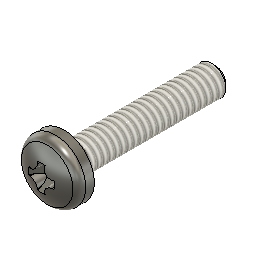
Airmote (Autodesk Fusion 360 archive; units mm, degrees)
design "Type I Cross Recessed Pan Head Machine Screw ANSI B18.6.7M M2x0.4 x 10 Steel Grade 2 Plain"
description: Type I Cross Recessed Pan Head Machine Screw ANSI B18.6.7M M2x0.4 x 10
part number: CRPHMSTI ANSI B18.6.7M - M2x0.4 x 10 Steel Grade 2 Plain
Autodesk Fusion 360 part; units mm, degrees
sketch "Sketch1" plane through (0, 0, 0) normal (0, 1, 0) x (1, 0, 0)
  line L0 (-1, 0) -> (-1, 10)
  line L1 (-1, 10) -> (0, 10)
  line L2 (0, 10) -> (0, -1.6)
  line L3 (-1, 0) -> (-2, 0)
  line L4 (-2, 0) -> (-2, -0.898)
  arc A0 (-2, -0.898) -> (0, -1.6) centre (0, 1.6) ccw
  dimension "d9" = 2
  dimension "d66" = 4
  dimension "d99" = 1.6
  dimension "d100" = 10
  constraint perpendicular L0 L1
  constraint perpendicular L0 L3
  constraint coincident origin L3
  constraint vertical L0
  constraint vertical L2
  constraint parallel L2 L4
  constraint coincident L2 A0.centre
  constraint coincident origin L2
  measures "d99" distance of L2.end L3
  measures "d100" distance of origin L1
revolve "Revolve1" add sketch "Sketch1" angle 360 about axis through (0, 0, -10) along (0, 0, 1) makes body 1
ref_plane "WorkPlane1" through (0, 0, 1.6) normal (0, 0, 1) x (1, 0, 0)
sketch "Sketch2" plane through (0, 0, 1.6) normal (0, 0, 1) x (1, 0, 0)
  line L0 (-0.24, 0.24) -> (-0.91, 0.24)
  line L1 (-0.24, -0.24) -> (-0.91, -0.24)
  line L2 (-0.91, 0.24) -> (-0.91, -0.24)
  line L3 (-0.24, -0.24) -> (-0.24, -0.91)
  line L4 (-0.24, -0.91) -> (0.24, -0.91)
  line L5 (0.24, -0.24) -> (0.24, -0.91)
  line L6 (0.24, -0.24) -> (0.91, -0.24)
  line L7 (0.91, -0.24) -> (0.91, 0.24)
  line L8 (0.24, 0.24) -> (0.91, 0.24)
  line L9 (0.24, 0.24) -> (0.24, 0.91)
  line L10 (0.24, 0.91) -> (-0.24, 0.91)
  line L11 (-0.24, 0.24) -> (-0.24, 0.91)
  dimension "d94" = 360
  dimension "d102" = 0.48
  dimension "d103" = 1.82
  constraint vertical L0.start L1.start
  constraint horizontal L0
  constraint coincident L0.start L11.start
  constraint vertical L2
  measures "d102" distance of L0 L1
  measures "d103" distance of L2 L7
extrude "Extrude1" add sketch "Sketch2" against normal blind 1.34 draft -4 separate body makes body 2
draft "Draft1" angle -30 neutral plane through (0, 0, 1.6) pull (0, 0, 1) 4 faces at (-0.8788, -0.0488, 1.1533) (0.0488, -0.8788, 1.1533) (0.8788, 0.0488, 1.1533) (-0.0488, 0.8788, 1.1533) on bodies 2
fillet "Fillet3" radius 0.48 4 edges at (-0.1931, 0.1931, 0.93) (0.1931, 0.1931, 0.93) (0.1931, -0.1931, 0.93) (-0.1931, -0.1931, 0.93) on bodies 2
combine "Combine1" operation cut target body 1 tool bodies 2
fillet "Fillet4" radius 0.64 1 edges at (-1.8647, 0.7232, 0.898) on bodies 1
thread "Thread3" "ANSI Metric M Profile 2.0 M2x0.4 M2x0.4 6g" major diameter 1.9335 minor diameter 1.478 pitch 0.4 angle 60 resizes the face on face at (-0.995, 0.0996, -6.6667) from (0, 0, -0.8) to (0, 0, -10) on bodies 1
sketch "Sketch5" plane through (0, 0, 0) normal (0, 1, 0) x (1, 0, 0)
  line L0 (-1.02, 10) -> (-1.02, 9.665)
  line L1 (-1.02, 9.665) -> (-0.665, 10)
  line L2 (0, 10) -> (0, -1.6)
  line L3 (-1.02, 10) -> (0, 10)
  dimension "d104" = 1.02
  dimension "d105" = 0.335
  dimension "d106" = 0.355
  constraint coincident L2.start L3.end
  constraint perpendicular L2 L3
  constraint coincident L1.end L3
  constraint perpendicular L0 L3
  measures "d104" distance of L0 L2.start
  measures "d105" distance of L0.end L3
  measures "d106" distance of L0 L1.end
revolve "Revolve2" cut sketch "Sketch5" angle 360 about axis through (0, 0, -10) along (0, 0, 1) bodies 1
equation "d9 = adsk_nomdia"
equation "adsk_nomlen = 10.00 mm"
equation "adsk_headh = 1.60 mm"
equation "adsk_headdia = 4.00 mm"
equation "adsk_nomdia = 2.00 mm"
equation "adsk_phildia = 1.82 mm"
equation "d31 = -adsk_phildepth"
equation "adsk_philwidth = 0.48 mm"
equation "adsk_phildepth = 1.34 mm"
equation "d66 = adsk_headdia"
equation "d71 = adsk_headh"
equation "adsk_thrlen = 9.20 mm"
equation "d76 = adsk_headtoprad"
equation "adsk_endpointdia = 1.33 mm"
equation "adsk_startlen = 0.335 mm"
equation "adsk_ovalrad = 3.20 mm"
equation "adsk_headtoprad = 0.64 mm"
equation "d98 = adsk_philwidth"
equation "d99 = adsk_headh"
equation "d100 = adsk_nomlen"
equation "d101 = ( adsk_nomlen + adsk_headh ) - ( adsk_ovalrad )"
equation "d102 = adsk_philwidth"
equation "d103 = adsk_phildia"
equation "d104 = adsk_nomdia * 0.51"
equation "d105 = adsk_startlen"
equation "d106 = ( adsk_nomdia * 0.51 ) - ( adsk_endpointdia / 2 )"
equation "d108 = min(adsk_thrlen; adsk_nomlen - 0.001 mm)"
